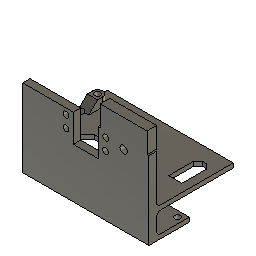
Flysky Screen Adapter (Autodesk Fusion 360 design; units mm, degrees)
part number: 2026-05-06-10-55-02-240
Autodesk Fusion 360 part; units mm, degrees
note: some values were not read from the file. Set by a fixed rule: which sketch regions a step uses.
sketch "Sketch1" plane through (0, 0, 0) normal (0, 0, 1) x (1, 0, 0)
  line L0 (0, 0) -> (86, 0)
  line L1 (86, 0) -> (86, 5)
  line L2 (86, 5) -> (0, 5)
  line L3 (0, 5) -> (0, 0)
  line L4 (43, 0) -> (51.5, 0)
  line L5 (51.5, 0) -> (51.5, 5)
  line L6 (51.5, 5) -> (43, 5)
  line L7 (43, 5) -> (43, 0) construction
  line L8 (43, 0) -> (34.5, 0)
  line L9 (34.5, 0) -> (34.5, 5)
  line L10 (34.5, 5) -> (43, 5)
  line L11 (43, 5) -> (43, 0) construction
  line L12 (0, 2.5) -> (86, 2.5) construction
  line L13 (86, 2.5) -> (86, 27.5)
  line L14 (86, 27.5) -> (0, 27.5)
  line L15 (0, 27.5) -> (0, 2.5)
  line L16 (0, 2.5) -> (86, 2.5) construction
  line L17 (86, 2.5) -> (86, -17.5)
  line L18 (86, -17.5) -> (0, -17.5)
  line L19 (0, -17.5) -> (0, 2.5)
  dimension "d1" = 86
  dimension "d2" = 5
  dimension "d3" = 8.5
  dimension "d4" = 8.5
  dimension "d5" = 25
  dimension "d6" = 20
  constraint horizontal L0
  constraint vertical L1
  constraint horizontal L2
  constraint vertical L3
  constraint coincident L0.start L3.end
  constraint horizontal L4
  constraint vertical L5
  constraint horizontal L6
  constraint vertical L7
  constraint midpoint L0 L4.start
  constraint horizontal L8
  constraint vertical L9
  constraint horizontal L10
  constraint vertical L11
  constraint horizontal L12
  constraint vertical L13
  constraint horizontal L14
  constraint vertical L15
  constraint midpoint L3 L12.start
  constraint horizontal L16
  constraint vertical L17
  constraint horizontal L18
  constraint vertical L19
  constraint coincident L2.end L10
  constraint coincident L2.end L6
  measures "d1" distance of L0.start L0.end
  measures "d2" distance of L0.start L2.end
  measures "d3" distance of L4.start L4.end
  measures "d4" distance of L4.start L8.end
  measures "d5" distance of L12.start L14.end
  measures "d6" distance of L12.start L18.end
extrude "Extrude1" add sketch "Sketch1" along normal blind 50 contours L0 L2 L3 L9 L15 L19 | L0 L1 L2 L5 L13 L17 makes body 1 at (74.5, 5, 16.6667) makes body 2 at (23, 5, 16.6667)
extrude "Extrude2" add sketch "Sketch1" against normal blind 3 contours L0 L2 L3 L9 L15 L19 | L0 L2 L4 L5 L6 L8 L9 L10 | L2 L6 L10 L13 L14 L15 | L0 L1 L2 L5 L13 L17 bodies 1 2
extrude "Extrude3" add sketch "Sketch1" along normal blind 3 from surface at 14 contours L2 L6 L10 L13 L14 L15 bodies 1
extrude "Extrude4" add sketch "Sketch1" along normal blind 31 contours L0 L2 L4 L5 L6 L8 L9 L10 bodies 1
sketch "Sketch2" plane through (0, 5, 0) normal (0, 1, 0) x (-1, 0, 0)
  line L0 (-86, 17) -> (0, 17)
  line L1 (0, 17) -> (0, 50)
  line L2 (0, 50) -> (-34.5, 50)
  line L3 (-34.5, 50) -> (-34.5, 31)
  line L4 (-34.5, 31) -> (-51.5, 31)
  line L5 (-51.5, 31) -> (-51.5, 50)
  line L6 (-51.5, 50) -> (-86, 50)
  line L7 (-86, 50) -> (-86, 17)
  line L8 (-68.75, 50) -> (-68.75, 45) construction
  circle A0 centre (-68.75, 45) radius 2.5
  line L9 (-51.5, 50) -> (-56.5, 50) construction
  line L10 (-56.5, 50) -> (-56.5, 46) construction
  line L11 (-56.5, 46) -> (-51.5, 46) construction
  line L12 (-51.5, 46) -> (-51.5, 50) construction
  line L13 (-34.5, 50) -> (-29.5, 50) construction
  line L14 (-29.5, 50) -> (-29.5, 46) construction
  line L15 (-29.5, 46) -> (-34.5, 46) construction
  line L16 (-34.5, 46) -> (-34.5, 50) construction
  circle A1 centre (-56.5, 46) radius 2
  circle A2 centre (-29.5, 46) radius 2
  line L17 (-29.5, 46) -> (-29.5, 38) construction
  line L18 (-56.5, 46) -> (-56.5, 38) construction
  circle A3 centre (-56.5, 38) radius 2
  circle A4 centre (-29.5, 38) radius 2
  line L19 (-68.75, 50) -> (-84.75, 50) construction
  line L20 (-84.75, 50) -> (-52.75, 50)
  line L21 (-52.75, 50) -> (-52.75, 64)
  line L22 (-52.75, 64) -> (-84.75, 64)
  line L23 (-84.75, 64) -> (-84.75, 50)
  dimension "d16" = 5
  dimension "d17" = 5
  dimension "d52" = 5
  dimension "d53" = 4
  dimension "d54" = 5
  dimension "d55" = 4
  dimension "d71" = 4
  dimension "d72" = 4
  dimension "d73" = 8
  dimension "d74" = 8
  dimension "d75" = 4
  dimension "d76" = 4
  dimension "d77" = 16
  dimension "d78" = 32
  dimension "d79" = 14
  constraint midpoint L6 L8.start
  constraint perpendicular L4 L8
  constraint coincident L8.end A0.centre
  constraint horizontal L9
  constraint vertical L10
  constraint horizontal L11
  constraint vertical L12
  constraint coincident L5.end L6.start
  constraint horizontal L13
  constraint vertical L14
  constraint horizontal L15
  constraint vertical L16
  constraint coincident L2.end L3.start
  constraint coincident L10.end L11.start
  constraint coincident L14.end L15.start
  constraint perpendicular L15 L17
  constraint perpendicular L11 L18
  constraint coincident L18.end A3.centre
  constraint coincident L17.end A4.centre
  constraint perpendicular L8 L19
  constraint horizontal L20
  constraint vertical L21
  constraint horizontal L22
  constraint vertical L23
  measures "d16" distance of L8.start L8.end
  measures "d17" diameter of A0
  measures "d52" distance of L5.end L9.end
  measures "d53" distance of L5.end L11.end
  measures "d54" distance of L2.end L13.end
  measures "d55" distance of L2.end L15.end
  measures "d71" diameter of A1
  measures "d72" diameter of A2
  measures "d73" distance of L14.end L17.end
  measures "d74" distance of L10.end L18.end
  measures "d75" diameter of A3
  measures "d76" diameter of A4
  measures "d77" distance of L8.start L19.end
  measures "d78" distance of L19.end L20.end
  measures "d79" distance of L19.end L22.end
extrude "Extrude5" cut sketch "Sketch2" against normal blind 5 contours A0 | A1 | A2 | A3 | A4 bodies 1
extrude "Extrude6" add 1 faces at (57.3333, 27.5, 15) along direction (0, 1, 0) blind 30 on bodies 1 bodies 1
sketch "Sketch3" plane through (0, 0, 17) normal (0, 0, 1) x (-1, 0, 0)
  line L0 (-86, -5) -> (-86, -57.5)
  line L1 (-86, -57.5) -> (0, -57.5)
  line L2 (0, -57.5) -> (0, -5)
  line L3 (0, -5) -> (-86, -5)
  line L4 (0, -5) -> (-54, -5)
  line L5 (-54, -5) -> (-54, -52)
  line L6 (-54, -52) -> (0, -52)
  line L7 (0, -52) -> (0, -5)
  line L8 (-54, -5) -> (-51, -5) construction
  line L9 (-51, -5) -> (-51, -8) construction
  line L10 (-51, -8) -> (-54, -8) construction
  line L11 (-54, -8) -> (-54, -5) construction
  circle A0 centre (-51, -8) radius 2
  line L12 (0, -52) -> (-5, -52) construction
  line L13 (-5, -52) -> (-5, -46) construction
  line L14 (-5, -46) -> (0, -46) construction
  line L15 (0, -46) -> (0, -52) construction
  circle A1 centre (-5, -46) radius 2
  circle A2 centre (-5, -46) radius 3.5
  circle A3 centre (-51, -8) radius 3.5
  line L16 (-54, -19) -> (-14, -19)
  line L17 (-54, -5) -> (-42, -5)
  line L18 (-42, -5) -> (-14, -5)
  line L19 (-14, -5) -> (-14, -19)
  line L20 (-14, -19) -> (-42, -19)
  line L21 (-42, -19) -> (-42, -5)
  line L22 (-5, -46) -> (-8.5, -46) construction
  line L23 (-8.5, -46) -> (-8.5, -42.5) construction
  line L24 (-8.5, -42.5) -> (-5, -42.5) construction
  line L25 (-5, -42.5) -> (-5, -46) construction
  line L26 (-8.5, -42.5) -> (-1.5, -42.5)
  line L27 (-1.5, -42.5) -> (-1.5, -46)
  line L28 (-1.5, -46) -> (-8.5, -46) construction
  line L29 (-8.5, -46) -> (-8.5, -42.5)
  line L30 (-54, -38) -> (-76, -38) construction
  line L31 (-80.5, -28) -> (-71.5, -28)
  line L32 (-71.5, -28) -> (-71.5, -48)
  line L33 (-71.5, -48) -> (-80.5, -48)
  line L34 (-80.5, -48) -> (-80.5, -28)
  line L35 (-80.5, -28) -> (-71.5, -48) construction
  line L36 (-71.5, -28) -> (-80.5, -48) construction
  line L37 (-54.5, -8.0076) -> (-54.5, -5.0076) construction
  line L38 (-54.5, -5.0076) -> (-47.5, -5.0076)
  line L39 (-47.5, -5.0076) -> (-47.5, -8.0076)
  line L40 (-47.5, -8.0076) -> (-54.5, -8.0076)
  line L41 (-54.5, -8.0076) -> (-54.5, -5.0076)
  point P0 (-76, -38)
  dimension "d22" = 54
  dimension "d23" = 47
  dimension "d24" = 3
  dimension "d25" = 3
  dimension "d26" = 4
  dimension "d27" = 5
  dimension "d28" = 6
  dimension "d29" = 4
  dimension "d30" = 7
  dimension "d31" = 7
  dimension "d34" = 40
  dimension "d35" = 12
  dimension "d36" = 14
  dimension "d39" = 3.5
  dimension "d40" = 3.5
  dimension "d41" = 22
  dimension "d42" = 9
  dimension "d43" = 20
  dimension "d84" = 14
  dimension "d98" = 3
  dimension "d99" = 3
  constraint horizontal L4
  constraint vertical L5
  constraint horizontal L6
  constraint vertical L7
  constraint coincident L2.end L3.start
  constraint horizontal L8
  constraint vertical L9
  constraint horizontal L10
  constraint vertical L11
  constraint coincident L9.end L10.start
  constraint horizontal L12
  constraint vertical L13
  constraint horizontal L14
  constraint vertical L15
  constraint coincident L13.end L14.start
  constraint concentric A1 A2
  constraint coincident L5 L16.start
  constraint perpendicular L5 L16
  constraint coincident L5 L4.end
  constraint perpendicular L5 L17
  constraint horizontal L18
  constraint vertical L19
  constraint horizontal L20
  constraint vertical L21
  constraint coincident L4.end L17
  constraint horizontal L22
  constraint vertical L23
  constraint horizontal L24
  constraint vertical L25
  constraint horizontal L26
  constraint vertical L27
  constraint horizontal L28
  constraint vertical L29
  constraint coincident A2 L27.end
  constraint coincident L14 L27.end
  constraint perpendicular L0 L30
  constraint horizontal L31
  constraint perpendicular L31 L32
  constraint parallel L31 L33
  constraint parallel L32 L34
  constraint coincident L35 P0
  constraint coincident L36 P0
  constraint coincident P0 L30.end
  constraint coincident L5 L30.start
  constraint coincident A3 L37.start
  constraint vertical L37
  constraint horizontal L38
  constraint vertical L39
  constraint horizontal L40
  constraint vertical L41
  constraint tangent A3 L39
  measures "d22" distance of L2.end L4.end
  measures "d23" distance of L2.end L6.end
  measures "d24" distance of L4.end L8.end
  measures "d25" distance of L4.end L10.end
  measures "d26" diameter of A0
  measures "d27" distance of L6.end L12.end
  measures "d28" distance of L6.end L14.end
  measures "d29" diameter of A1
  measures "d30" diameter of A2
  measures "d31" diameter of A3
  measures "d34" distance of L16.start L16.end
  measures "d35" distance of L4.end L17.end
  measures "d36" distance of L4 L16
  measures "d39" distance of L13.end L22.end
  measures "d40" distance of L13.end L24.end
  measures "d41" distance of L30.start P0
  measures "d42" distance of L32.end L33.end
  measures "d43" distance of L31.end L32.end
  measures "d84" distance of L6 L30
  measures "d98" distance of L37.start L37.end
  measures "d99" distance of L37.end L37.start
extrude "Extrude7" add sketch "Sketch3" along normal blind 6 contours L5 A3 L38 L41 | L3 L4 A3 L17 L38 | L5 A3 L38 | L5 A0 A3 L38 L39 L40 | L5 A3 L40 | A3 L38 L39 | L5 A0 A3 L40 | L5 A3 L40 | A2 | A2 L26 L29 | A2 L26 L27 bodies 1
extrude "Extrude8" cut sketch "Sketch3" against normal blind 3 contours L3 L4 L16 L18 L19 L20 L21 | L31 L32 L33 L34 bodies 1
sketch "Sketch4" plane through (0, 0, -3) normal (0, 0, -1) x (1, 0, 0)
  line L0 (86, -27.5) -> (86, 0)
  line L1 (86, 0) -> (0, 0)
  line L2 (0, 0) -> (0, -27.5)
  line L3 (0, -27.5) -> (86, -27.5)
  line L4 (86, -27.5) -> (82, -27.5) construction
  line L5 (82, -27.5) -> (82, -23.5) construction
  line L6 (82, -23.5) -> (86, -23.5) construction
  line L7 (86, -23.5) -> (86, -27.5) construction
  circle A0 centre (82, -23.5) radius 2
  line L8 (0, -27.5) -> (4, -27.5) construction
  line L9 (4, -27.5) -> (4, -23.5) construction
  line L10 (4, -23.5) -> (0, -23.5) construction
  line L11 (0, -23.5) -> (0, -27.5) construction
  circle A1 centre (4, -23.5) radius 2
  line L12 (4, -23.5) -> (44, -23.5) construction
  circle A2 centre (44, -23.5) radius 2
  circle A3 centre (4, -35.5) radius 2
  circle A4 centre (44, -35.5) radius 2
  dimension "d44" = 4
  dimension "d45" = 4
  dimension "d86" = 4
  dimension "d87" = 4
  dimension "d88" = 4
  dimension "d89" = 4
  dimension "d90" = 40
  dimension "d91" = 4
  dimension "d94" = 0
  dimension "d95" = -12
  constraint horizontal L4
  constraint vertical L5
  constraint horizontal L6
  constraint vertical L7
  constraint coincident L0.start L3.end
  constraint coincident L5.end L6.start
  constraint horizontal L8
  constraint vertical L9
  constraint horizontal L10
  constraint vertical L11
  constraint coincident L2.end L3.start
  constraint coincident L9.end L10.start
  constraint perpendicular L9 L12
  constraint coincident L12.end A2.centre
  measures "d44" distance of L0.start L4.end
  measures "d45" distance of L0.start L6.end
  measures "d86" diameter of A0
  measures "d87" distance of L2.end L8.end
  measures "d88" distance of L2.end L10.end
  measures "d89" diameter of A1
  measures "d90" distance of L9.end L12.end
  measures "d91" diameter of A2
extrude "Extrude9" cut sketch "Sketch4" against normal blind 3 contours A0 | A1 | A2 bodies 1
extrude "Extrude13" add sketch "Sketch2" along normal blind 1.5 and the other way blind 5 contours L6 L20 L21 L22 L23 bodies 1
chamfer "Chamfer1" distance 3 angle 45 2 edges at (80.5, 48, 15.5) (71.5, 48, 15.5) on bodies 1
extrude "Extrude14" cut sketch "Sketch4" against normal blind 20 contours A3 | A4 bodies 1
chamfer "Chamfer2" distance 6 angle 45 1 edges at (5, 42.5, 17) on bodies 1
extrude "Extrude15" cut 1 faces at (32.6667, 19, 16) along direction (0, 1, 0) blind 8 on bodies 1 bodies 1
chamfer "Chamfer3" distance 8 angle 45 2 edges at (42, 27, 15.5) (14, 27, 15.5) on bodies 1
chamfer "Chamfer4" distance 2 angle 45 6 edges at (43, 5, 0) (7, 5, 14) (64, 5, 14) (45.5986, 5, 17) (69.4014, 5, 17) (7, 5, 17) on bodies 1
